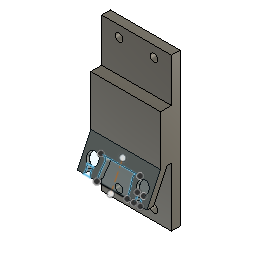
holder (Autodesk Fusion 360 design; units mm, degrees)
Autodesk Fusion 360 part; units mm, degrees
note: some values were not read from the file. Set by a fixed rule: which sketch regions a step uses.
sketch "Skizze1" plane through (0, 0, 0) normal (1, 0, 0) x (0, 1, 0)
  line L0 (7, 50) -> (7, -20)
  line L1 (-9.0346, 36) -> (15, -14) construction
  line L2 (-5.2641, -6.0314) -> (1, 7)
  line L3 (-2, 7) -> (-8.2641, -6.0314)
  line L4 (-8.2641, -6.0314) -> (-5.2641, -6.0314)
  line L5 (-2, 7) -> (-2, 30)
  line L6 (7, -20) -> (3, -20)
  line L7 (3, -20) -> (3, 7)
  line L8 (3, 7) -> (1, 7)
  line L9 (7, 50) -> (3, 50)
  line L10 (3, 50) -> (3, 30)
  line L11 (3, 30) -> (-2, 30)
  constraint vertical L0
  constraint perpendicular L0 L6
  constraint perpendicular L6 L7
  constraint perpendicular L7 L8
  constraint perpendicular L0 L9
  constraint perpendicular L9 L10
extrude "Extrusion2" add sketch "Skizze1" along normal mid plane 32
sketch "Skizze7" plane through (0, -1.921, 0.9234) normal (0, 0.90128, -0.433238) x (-1, 0, 0)
  circle A0 centre (11.5, -3) radius 3.5
  circle A1 centre (-11.5, -3) radius 2.75
  line L0 (-16, 6.7422) -> (-16, -7.7165)
  line L1 (-16, -7.7165) -> (16, -7.7165)
  line L2 (16, -7.7165) -> (16, 6.7422)
  circle A2 centre (-11.5, -3) radius 3.5
  circle A3 centre (11.5, -3) radius 2.75
  line L3 (16, 6.7422) -> (-16, 6.7422)
  dimension "d19" = 7
  dimension "d20" = 5.5
  dimension "d43" = 7
  dimension "d44" = 5.5
  measures "d19" diameter of A0
  measures "d20" diameter of A1
  measures "d43" diameter of A2
  measures "d44" diameter of A3
extrude "Extrusion9" cut sketch "Skizze7" against normal blind 3 contours A1 | A3
extrude "Extrusion15" cut sketch "Skizze7" against normal blind 1 contours A0 | A2
sketch "Skizze11" plane through (0, 7, 0) normal (0, 1, 0) x (-1, 0, 0)
  line L0 (-16, 50) -> (-16, -20)
  line L1 (-16, -20) -> (16, -20)
  line L2 (16, -20) -> (16, 50)
  circle A0 centre (-8, 45) radius 1.75
  circle A1 centre (8, 45) radius 1.75
  circle A2 centre (-8, 25) radius 1.75
  circle A3 centre (8, 25) radius 1.75
  circle A4 centre (-8, 5) radius 1.75
  circle A5 centre (8, 5) radius 1.75
  line L3 (16, 50) -> (-16, 50)
  circle A6 centre (8, -15) radius 1.75
  circle A7 centre (-8, -15) radius 1.75
  dimension "d47" = 3.5
  dimension "d48" = 3.5
  dimension "d49" = 3.5
  dimension "d50" = 3.5
  dimension "d51" = 3.5
  dimension "d52" = 3.5
  dimension "d53" = 3.5
  dimension "d54" = 3.5
  measures "d47" diameter of A0
  measures "d48" diameter of A1
  measures "d49" diameter of A2
  measures "d50" diameter of A3
  measures "d51" diameter of A4
  measures "d52" diameter of A5
  measures "d53" diameter of A7
  measures "d54" diameter of A6
extrude "Extrusion16" cut sketch "Skizze11" against normal blind 4 contours A0 | A1 | A2 | A3 | A4 | A5 | A6 | A7
sketch "Skizze12" plane through (0, -4.3579, 2.0948) normal (0, -0.90128, 0.433238) x (1, 0, 0)
  circle A0 centre (-11.5, -3) radius 2.75
  circle A1 centre (11.5, -3) radius 2.75
  line L0 (-16, -9.0163) -> (16, -9.0163)
  line L1 (16, -9.0163) -> (16, 5.4425)
  line L2 (16, 5.4425) -> (-16, 5.4425)
  line L3 (-16, 5.4425) -> (-16, -9.0163)
  line L4 (10.0325, -9.0163) -> (10.5, -7)
  line L5 (10.5, -7) -> (10.0325, -5.3257)
  line L6 (12.9675, -5.3257) -> (12.5, -7)
  line L7 (12.5, -7) -> (13.0021, -9.0163)
  line L8 (10.0325, -9.0163) -> (13.0021, -9.0163)
  line L9 (10.0325, -5.3257) -> (12.9675, -5.3257)
  line L10 (9, 0) -> (-9, 0)
  line L11 (-6.9785, -9.0163) -> (7, -9.0163)
  line L12 (0, 2.4733) -> (0, -10.3438) construction
  line L13 (-10.0325, -5.3257) -> (-12.9675, -5.3257)
  line L14 (-10.5, -7) -> (-10.0325, -5.3257)
  line L15 (-10.0325, -9.0163) -> (-10.5, -7)
  line L16 (-10.0325, -9.0163) -> (-13.0021, -9.0163)
  line L17 (-12.5, -7) -> (-13.0021, -9.0163)
  line L18 (-12.9675, -5.3257) -> (-12.5, -7)
  spline S0 degree 5 poles (-9, 0) (-8.4547, 0) (-7.5256, -0.0717) (-6.6164, -0.3941) (-6.2178, -1.2222) (-6.4705, -2.8946) (-6.8177, -4.8332) (-6.9655, -6.7297) (-6.987, -8.2169) (-6.9785, -9.0163) knots 0 0 0 0 0 0 0.2 0.4 0.6 0.8 1 1 1 1 1 1
  spline S1 degree 5 poles (7, -9.0163) (7, -8.2162) (6.9641, -6.7278) (6.8026, -4.8304) (6.4506, -2.8919) (6.2043, -1.2206) (6.6105, -0.3936) (7.5237, -0.0716) (8.4542, 0) (9, 0) knots 0 0 0 0 0 0 0.2 0.4 0.6 0.8 1 1 1 1 1 1
  line L19 (-10, 0) -> (-8, 0)
  line L20 (8, 0) -> (10, 0)
  line L21 (-7, -7) -> (-6.957, -11.0325)
  line L22 (7, -11.0325) -> (7, -7)
  constraint coincident L0 L4.start
  constraint coincident A1 L5.end
  constraint coincident A1 L6.start
  constraint coincident L0 L7.end
  constraint parallel L8 L9
  constraint horizontal L10
  constraint horizontal L11
  constraint coincident L0 L11.start
  constraint perpendicular L0 L12
  constraint symmetric L4.start L12 L15.start
  constraint symmetric L4.end L12 L14.start
  constraint symmetric L5.end L12 L13.start
  constraint symmetric L6.start L12 L13.end
  constraint symmetric L6.end L12 L17.start
  constraint symmetric L7.end L12 L16.end
  constraint midpoint L10.end L19
  constraint midpoint L10.start L20
  constraint midpoint L11.start L21
  constraint midpoint L11.end L22
  constraint coincident L10 L20.start
extrude "Extrusion17" cut sketch "Skizze12" against normal blind 2.8 contours A0 L0 L14 L15 L16 L17 L18 | L0 L10 L11 S0 S1 L19 L20 | A1 L0 L4 L5 L6 L7 L8
